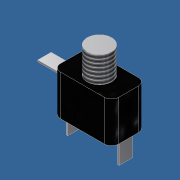
# Autodesk Inventor part: P1704_002_picotte_alexandre
Saved by Autodesk Inventor 2015 SP2 (Build 190223200, 223)
## iProperties
Created: 2018-05-04
Part Number: P1704_002_picotte_alexandre
Project: Nom Projet
Material: .
Description: Nom pièce
Document SubType Name: Modeling
Designer: Alexandre.PICOTTE
Authority: brut Ø
Density: 0.001 g/cm^3
Appearance: Noir
Material number: ---
Author: Alexandre.PICOTTE
Autodesk Inventor part; units mm, degrees
ref_plane "Plan YZ" through (0, 0, 0) normal (1, 0, 0) x (0, 1, 0)
ref_plane "Plan XZ" through (0, 0, 0) normal (0, 1, 0) x (-1, 0, 0)
ref_plane "Plan XY" through (0, 0, 0) normal (0, 0, 1) x (1, 0, 0)
sketch "Esquisse1" plane through (0, 0, 0) normal (0, 0, 1) x (1, 0, 0)
  line L0 (-10.45, 8.165) -> (10.45, 8.165)
  line L1 (13.95, 4.665) -> (13.95, -4.665)
  line L2 (10.45, -8.165) -> (-10.45, -8.165)
  line L3 (-13.95, -4.665) -> (-13.95, 4.665)
  line L4 (-20.5448, 0) -> (20.5448, 0) construction
  line L5 (0, -12.4458) -> (0, 12.4458) construction
  arc A0 (-10.45, 8.165) -> (-13.95, 4.665) centre (-10.45, 4.665) ccw
  arc A1 (13.95, 4.665) -> (10.45, 8.165) centre (10.45, 4.665) ccw
  arc A2 (10.45, -8.165) -> (13.95, -4.665) centre (10.45, -4.665) ccw
  arc A3 (-13.95, -4.665) -> (-10.45, -8.165) centre (-10.45, -4.665) ccw
  point P0 (0, 0)
  point P1 (-13.95, 8.165)
  point P2 (13.95, 8.165)
  point P3 (-13.95, -8.165)
  dimension "d0" = 16.33
  dimension "d1" = 27.9
  dimension "d2" = 3.5
  constraints: 8 end point, 8 point on circle, 8 tangent, 6 point on line, 4 centre point, 3 equal radius, 2 parallel, 1 horizontal, 1 perpendicular, 2 other
  measures "d0" distance of point (-13.95, -8.165) point (-13.95, 8.165)
  measures "d1" distance of point (-13.95, 8.165) point (13.95, 8.165)
  measures "d2" radius of A0
extrude "Extrusion1" add sketch "Esquisse1" along normal blind 19.3
sketch "Esquisse6" plane through (0, 0, 19.3) normal (0, 0, 1) x (1, 0, 0)
  circle A0 centre (0, 0) radius 5.835
  dimension "d5" = 11.67
  constraints: 1 centre point, 1 coincident
  measures "d5" diameter of A0
extrude "Extrusion2" add sketch "Esquisse6" along normal blind 12.45
thread "Filetage1" size "M12x1.75" class "6g" standard "ISO M" full length
sketch "Esquisse7" plane through (0, 0, 0) normal (0, 0, -1) x (-1, 0, 0)
  line L0 (0, -11.431) -> (0, 11.431) construction
  line L1 (19.53, 0) -> (-19.53, 0) construction
  line L2 (12.65, -3.2) -> (11.89, -3.2)
  line L3 (11.89, -3.2) -> (11.89, 3.2)
  line L4 (11.89, 3.2) -> (12.65, 3.2)
  line L5 (12.65, 3.2) -> (12.65, -3.2)
  line L6 (-11.89, -3.2) -> (-12.65, -3.2)
  line L7 (-12.65, -3.2) -> (-12.65, 3.2)
  line L8 (-12.65, 3.2) -> (-11.89, 3.2)
  line L9 (-11.89, 3.2) -> (-11.89, -3.2)
  line L10 (13.95, -4.665) -> (13.95, 4.665) construction
  point P0 (0, 0)
  dimension "d10" = 1.3
  dimension "d11" = 0.76
  dimension "d12" = 6.4
  constraints: 16 end point, 4 parallel, 2 horizontal, 2 perpendicular, 5 other
  measures "d10" distance between parallel lines of L10 L5
  measures "d11" distance of L2.start L2.end
  measures "d12" distance of L4.end L2.start
extrude "Extrusion3" add sketch "Esquisse7" along normal blind 10.25
sketch "Esquisse8" plane through (-13.95, -4.665, 0) normal (-1, 0, 0) x (0, 0, 1)
  line L0 (16.45, 4.55) -> (17.21, 4.55)
  line L1 (17.21, 4.55) -> (17.21, -1.85)
  line L2 (17.21, -1.85) -> (16.45, -1.85)
  line L3 (16.45, -1.85) -> (16.45, 4.55)
  line L4 (19.3, 9.33) -> (19.3, 0) construction
  line L5 (0, -3.5) -> (19.3, -3.5) projected
  point P0 (0, 4.665)
  dimension "d15" = 2.85
  dimension "d16" = 0.76
  dimension "d17" = 6.4
  dimension "d18" = 1.65
  constraints: 8 end point, 2 parallel, 1 horizontal, 1 perpendicular
  measures "d15" distance between parallel lines of L4 L3
  measures "d16" distance of L1.end L2.end
  measures "d17" distance of L0.end L1.end
  measures "d18" distance between parallel lines of L5 L2
extrude "Extrusion4" add sketch "Esquisse8" along normal blind 9
equation "\"d16\" = d11"
equation "\"d17\" = d12"
